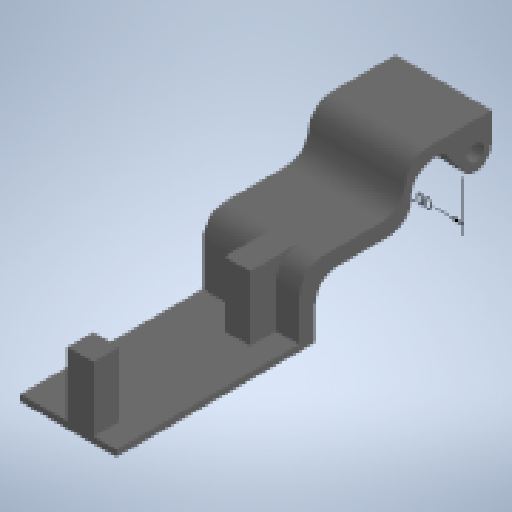
# Autodesk Inventor part: arm_0
Saved by Autodesk Inventor 2024.1 (Build 281209000, 209)
## iProperties
Created: 2025-01-27
Part Number: arm_0
Material: 一般
Document SubType Name: Modeling
Designer: hibik
Density: 1 g/cm^3
Appearance: 既定
Author: hibik
Autodesk Inventor part; units mm, degrees
ref_plane "YZ Plane" through (0, 0, 0) normal (1, 0, 0) x (0, 1, 0)
ref_plane "XZ Plane" through (0, 0, 0) normal (0, 1, 0) x (-1, 0, 0)
sketch "スケッチ1" plane through (0, 0, 0) normal (0, 1, 0) x (-1, 0, 0)
  line L0 (15, 0) -> (-15, 0)
  line L1 (-15, 0) -> (-15, -56.8)
  line L2 (-15, -56.8) -> (15, -56.8)
  line L3 (15, -56.8) -> (15, 0)
  point P0 (0, 0)
  point P1 (0, 0)
  dimension "d0" = 30
  dimension "d9" = 56.8
  constraints: 8 end point, 2 parallel, 1 coincident, 1 horizontal, 1 midpoint, 1 perpendicular
  measures "d0" distance of L0.start L0.end
  measures "d9" distance of L2.end L0.start
extrude "押し出し1" add sketch "スケッチ1" along normal blind 2
ref_plane "作業平面1" through (7.8, 0, 0) normal (1, 0, 0) x (0, 0, -1)
sketch "スケッチ2" plane through (7.8, 0, 0) normal (1, 0, 0) x (0, 0, -1)
  line L0 (0, 2) -> (56.8, 2)
  line L1 (56.8, 2) -> (56.8, 22.1)
  line L2 (56.8, 22.1) -> (0, 22.1)
  line L3 (0, 22.1) -> (0, 2)
  line L4 (8, 2) -> (48.8, 2)
  line L5 (48.8, 2) -> (48.8, 22.1)
  line L6 (48.8, 22.1) -> (8, 22.1)
  line L7 (8, 22.1) -> (8, 2)
  line L8 (0, 2) -> (56.8, 2) projected
  line L9 (0, 0) -> (0, 2) projected
  point P0 (28.4, 22.1)
  dimension "d4" = 56.8
  dimension "d5" = 40.8
  dimension "d6" = 20.1
  constraints: 16 end point, 4 parallel, 2 collinear, 2 horizontal, 2 midpoint, 2 perpendicular, 2 point on line
  measures "d4" distance of L2.end L1.end
  measures "d5" distance of L6.end L5.end
  measures "d6" distance of L2.end L0.start
extrude "押し出し2" add sketch "スケッチ2" against normal blind 8 contours L3 L2 L7 L0 | L5 L2 L1 L0
sketch "スケッチ3" plane through (15, 0, -56.8) normal (0, 0, -1) x (-1, 0, 0)
  line L0 (30, 0) -> (0, 0) projected
  line L1 (0, 0) -> (30, 0)
  line L2 (30, 0) -> (30, 22.1)
  line L3 (30, 22.1) -> (0, 22.1)
  line L4 (0, 22.1) -> (0, 0)
  line L5 (7.2, 22.1) -> (15.2, 22.1) projected
  line L6 (30, 0) -> (30, 2) projected
  point P0 (15, 0)
  constraints: 8 end point, 2 collinear, 2 parallel, 1 horizontal, 1 perpendicular
extrude "押し出し3" add sketch "スケッチ3" along normal blind 5
sketch "スケッチ4" plane through (15, 0, -61.8) normal (0, 0, -1) x (-1, 0, 0)
  line L0 (7.2, 22.1) -> (0, 22.1) projected
  line L1 (30, 2) -> (30, 22.1) projected
  line L2 (0, 22.1) -> (30, 22.1)
  line L3 (30, 22.1) -> (30, 17.1)
  line L4 (30, 17.1) -> (0, 17.1)
  line L5 (0, 17.1) -> (0, 22.1)
  point P0 (15, 0)
  point P1 (7.2, 22.1)
  dimension "d12" = 5
  constraints: 8 end point, 2 parallel, 1 horizontal, 1 perpendicular, 1 point on line
  measures "d12" distance of L2.end L3.end
extrude "押し出し4" add sketch "スケッチ4" along normal blind 28
sketch "スケッチ5" plane through (15, 0, -89.8) normal (0, 0, -1) x (-1, 0, 0)
  line L0 (0, 17.1) -> (30, 17.1) projected
  line L1 (0, 17.1) -> (30, 17.1)
  line L2 (30, 17.1) -> (30, 35.1)
  line L3 (30, 35.1) -> (0, 35.1)
  line L4 (0, 35.1) -> (0, 17.1)
  line L5 (30, 17.1) -> (30, 22.1) projected
  line L6 (30, 22.1) -> (0, 22.1) projected
  point P0 (15, 0)
  dimension "d21" = 13
  constraints: 8 end point, 2 parallel, 1 collinear, 1 horizontal, 1 perpendicular
  measures "d21" distance between parallel lines of L3 L6
extrude "押し出し5" add sketch "スケッチ5" along normal blind 2
sketch "スケッチ6" plane through (15, 0, -91.8) normal (0, 0, -1) x (-1, 0, 0)
  line L0 (30, 22.1) -> (30, 35.1) projected
  line L1 (0, 35.1) -> (30, 35.1)
  line L2 (30, 35.1) -> (30, 31.1)
  line L3 (30, 31.1) -> (0, 31.1)
  line L4 (0, 31.1) -> (0, 35.1)
  line L5 (0, 35.1) -> (0, 17.1) projected
  line L6 (30, 35.1) -> (0, 35.1) projected
  point P0 (15, 0)
  point P1 (30, 35.1)
  dimension "d18" = 4
  constraints: 8 end point, 2 collinear, 2 parallel, 1 horizontal, 1 perpendicular, 1 point on line
  measures "d18" distance between parallel lines of L1 L3
extrude "押し出し6" add sketch "スケッチ6" along normal blind 25
fillet "フィレット1" radius 7 7 edges at (0, 17.1, -61.8) (0, 17.1, -91.8) (0, 31.1, -91.8) (0, 22.1, -89.8) (0, 35.1, -89.8) (11.4, 22.1, -56.8) (-7.6, 22.1, -56.8)
sketch "スケッチ7" plane through (15, 0, 0) normal (1, 0, 0) x (0, 0, -1)
  circle A0 centre (111.8, 26.1) radius 5
  circle A1 centre (111.8, 26.1) radius 2.5
  line L0 (98.8, 31.1) -> (116.8, 31.1) projected
  line L1 (116.8, 35.1) -> (116.8, 31.1) projected
  line L2 (116.8, 31.1) -> (116.8, 26.1)
  line L3 (101.8, 31.1) -> (107.8, 23.1)
  point P0 (0, 0)
  dimension "d23" = 10
  dimension "d24" = 5
  dimension "d25" = 10
  constraints: 4 end point, 3 tangent, 2 centre point, 2 point on circle, 1 coincident, 1 point on line, 1 vertical
  measures "d23" diameter of A0
  measures "d24" diameter of A1
  measures "d25" horizontal distance of A0.centre L3.start
extrude "押し出し7" add sketch "スケッチ7" against normal up to surface (30 mm away)
